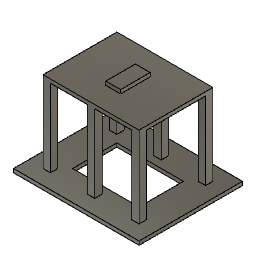
Project Stand v7 (Autodesk Fusion 360 design; units mm, degrees)
Autodesk Fusion 360 part; units mm, degrees
sketch "Sketch1" plane through (0, 0, 0) normal (0, 0, 1) x (1, 0, 0)
  line L0 (-17.3001, 65.9212) -> (152.6999, 65.9212)
  line L1 (152.6999, 65.9212) -> (152.6999, -74.0788)
  line L2 (152.6999, -74.0788) -> (-17.3001, -74.0788)
  line L3 (-17.3001, -74.0788) -> (-17.3001, 65.9212)
  dimension "d1" = 140
  dimension "d2" = 170
  constraint horizontal L0
  constraint vertical L1
  constraint horizontal L2
  constraint vertical L3
  measures "d1" distance of L0 L2
  measures "d2" distance of L1 L3
extrude "Extrude1" add sketch "Sketch1" along normal blind 5
sketch "Sketch6" plane through (0, 0, 5) normal (0, 0, 1) x (-1, 0, 0)
  line L0 (17.3001, 74.0788) -> (-152.6999, 74.0788)
  line L1 (-152.6999, 74.0788) -> (-152.6999, -65.9212)
  line L2 (-152.6999, -65.9212) -> (17.3001, -65.9212)
  line L3 (17.3001, -65.9212) -> (17.3001, 74.0788)
  line L4 (-2.6999, 54.0788) -> (-132.6999, 54.0788)
  line L5 (-132.6999, 54.0788) -> (-132.6999, -45.9212)
  line L6 (-132.6999, -45.9212) -> (-2.6999, -45.9212)
  line L7 (-2.6999, -45.9212) -> (-2.6999, 54.0788)
  line L8 (17.3001, 74.0788) -> (17.3001, -65.9212)
  line L9 (-152.6999, -65.9212) -> (-152.6999, 74.0788)
  line L10 (-152.6999, 74.0788) -> (17.3001, 74.0788)
  line L11 (17.3001, -65.9212) -> (-152.6999, -65.9212)
  line L12 (-2.6999, 54.0788) -> (-12.6999, 54.0788)
  line L13 (-12.6999, 54.0788) -> (-12.6999, 44.0788)
  line L14 (-12.6999, 44.0788) -> (-2.6999, 44.0788)
  line L15 (-2.6999, 44.0788) -> (-2.6999, 54.0788)
  line L16 (-2.6999, -45.9212) -> (-12.6999, -45.9212)
  line L17 (-12.6999, -45.9212) -> (-12.6999, -35.9212)
  line L18 (-12.6999, -35.9212) -> (-2.6999, -35.9212)
  line L19 (-2.6999, -35.9212) -> (-2.6999, -45.9212)
  line L20 (-132.6999, 54.0788) -> (-122.6999, 54.0788)
  line L21 (-122.6999, 54.0788) -> (-122.6999, 44.0788)
  line L22 (-122.6999, 44.0788) -> (-132.6999, 44.0788)
  line L23 (-132.6999, 44.0788) -> (-132.6999, 54.0788)
  line L24 (-132.6999, -45.9212) -> (-122.6999, -45.9212)
  line L25 (-122.6999, -45.9212) -> (-122.6999, -35.9212)
  line L26 (-122.6999, -35.9212) -> (-132.6999, -35.9212)
  line L27 (-132.6999, -35.9212) -> (-132.6999, -45.9212)
  line L28 (-62.6999, 54.0788) -> (-72.6999, 54.0788)
  line L29 (-72.6999, 54.0788) -> (-72.6999, 44.0788)
  line L30 (-72.6999, 44.0788) -> (-62.6999, 44.0788)
  line L31 (-62.6999, 44.0788) -> (-62.6999, 54.0788)
  line L32 (-62.6999, -45.9212) -> (-72.6999, -45.9212)
  line L33 (-72.6999, -45.9212) -> (-72.6999, -35.9212)
  line L34 (-72.6999, -35.9212) -> (-62.6999, -35.9212)
  line L35 (-62.6999, -35.9212) -> (-62.6999, -45.9212)
  line L36 (-22.6999, -25.9212) -> (-112.6999, -25.9212)
  line L37 (-112.6999, -25.9212) -> (-112.6999, 34.0788)
  line L38 (-112.6999, 34.0788) -> (-22.6999, 34.0788)
  line L39 (-22.6999, 34.0788) -> (-22.6999, -25.9212)
  dimension "d23" = 20
  dimension "d24" = 20
  dimension "d25" = 20
  dimension "d26" = 20
  dimension "d27" = 10
  dimension "d28" = 10
  dimension "d29" = 10
  dimension "d30" = 10
  dimension "d31" = 10
  dimension "d32" = 10
  dimension "d33" = 10
  dimension "d34" = 10
  dimension "d35" = 10
  dimension "d36" = 10
  dimension "d37" = 10
  dimension "d38" = 10
  dimension "d39" = 50
  dimension "d40" = 50
  dimension "d41" = 50
  dimension "d42" = 50
  dimension "d57" = 10
  dimension "d58" = 10
  dimension "d59" = 10
  dimension "d60" = 10
  dimension "d61" = 20
  dimension "d62" = 20
  constraint horizontal L4
  constraint vertical L5
  constraint horizontal L6
  constraint vertical L7
  constraint horizontal L12
  constraint vertical L13
  constraint horizontal L14
  constraint vertical L15
  constraint horizontal L16
  constraint vertical L17
  constraint horizontal L18
  constraint vertical L19
  constraint horizontal L20
  constraint vertical L21
  constraint horizontal L22
  constraint vertical L23
  constraint horizontal L24
  constraint vertical L25
  constraint horizontal L26
  constraint vertical L27
  constraint horizontal L28
  constraint vertical L29
  constraint horizontal L30
  constraint vertical L31
  constraint coincident L4 L28.start
  constraint horizontal L32
  constraint vertical L33
  constraint horizontal L34
  constraint vertical L35
  constraint coincident L6 L32.start
  constraint horizontal L36
  constraint vertical L37
  constraint horizontal L38
  constraint vertical L39
  measures "d23" distance of L7 L8
  measures "d24" distance of L5 L9
  measures "d25" distance of L4 L10
  measures "d26" distance of L6 L11
  measures "d27" distance of L12 L14
  measures "d28" distance of L13 L15
  measures "d29" distance of L6 L18
  measures "d30" distance of L17 L19
  measures "d31" distance of L21 L23
  measures "d32" distance of L4 L22
  measures "d33" distance of L25 L27
  measures "d34" distance of L6 L26
  measures "d35" distance of L4 L30
  measures "d36" distance of L6 L34
  measures "d37" distance of L29 L31
  measures "d38" distance of L33 L35
  measures "d39" distance of L13 L31
  measures "d40" distance of L21 L29
  measures "d41" distance of L17 L35
  measures "d42" distance of L25 L33
  measures "d57" distance of L18 L36
  measures "d58" distance of L14 L38
  measures "d59" distance of L26 L36
  measures "d60" distance of L22 L38
  measures "d61" distance of L7 L39
  measures "d62" distance of L5 L37
extrude "Extrude4" add sketch "Sketch6" along normal blind 105 contours L4 L7 L12 L13 L14 L15 | L4 L28 L29 L30 L31 | L6 L7 L16 L17 L18 L19 | L4 L5 L20 L21 L22 L23 | L6 L32 L33 L34 L35 | L5 L6 L24 L25 L26 L27
sketch "Sketch7" plane through (0, 0, 110) normal (0, 0, 1) x (-1, 0, 0)
  line L0 (-2.6999, 44.0788) -> (-2.6999, 54.0788)
  line L1 (-2.6999, 54.0788) -> (-12.6999, 54.0788)
  line L2 (-12.6999, 54.0788) -> (-12.6999, 44.0788)
  line L3 (-12.6999, 44.0788) -> (-2.6999, 44.0788)
  line L4 (-2.6999, 54.0788) -> (-132.6999, 54.0788)
  line L5 (-132.6999, 54.0788) -> (-132.6999, -45.9212)
  line L6 (-132.6999, -45.9212) -> (-2.6999, -45.9212)
  line L7 (-2.6999, -45.9212) -> (-2.6999, 54.0788)
  dimension "d45" = 130
  dimension "d46" = 100
  constraint horizontal L4
  constraint vertical L5
  constraint horizontal L6
  constraint vertical L7
  constraint coincident L0.end L1.start
  measures "d45" distance of L5 L7
  measures "d46" distance of L4 L6
extrude "Extrude5" add sketch "Sketch7" along normal blind 5
sketch "Sketch8" plane through (0, 0, 115) normal (0, 0, 1) x (-1, 0, 0)
  line L0 (-2.6999, -45.9212) -> (-2.6999, 54.0788)
  line L1 (-2.6999, 54.0788) -> (-132.6999, 54.0788)
  line L2 (-132.6999, 54.0788) -> (-132.6999, -45.9212)
  line L3 (-132.6999, -45.9212) -> (-2.6999, -45.9212)
  line L4 (-57.6999, -15.9212) -> (-77.6999, -15.9212)
  line L5 (-77.6999, -15.9212) -> (-77.6999, 24.0788)
  line L6 (-77.6999, 24.0788) -> (-57.6999, 24.0788)
  line L7 (-57.6999, 24.0788) -> (-57.6999, -15.9212)
  dimension "d49" = 40
  dimension "d50" = 20
  dimension "d51" = 55
  dimension "d52" = 55
  dimension "d53" = 30
  dimension "d54" = 30
  constraint horizontal L4
  constraint vertical L5
  constraint horizontal L6
  constraint vertical L7
  measures "d49" distance of L4 L6
  measures "d50" distance of L5 L7
  measures "d51" distance of L0 L7
  measures "d52" distance of L2 L5
  measures "d53" distance of L3 L4
  measures "d54" distance of L1 L6
extrude "Extrude6" add sketch "Sketch8" along normal blind 5 contours L4 L5 L6 L7
extrude "Extrude7" cut sketch "Sketch6" against normal blind 5 contours L36 L37 L38 L39
